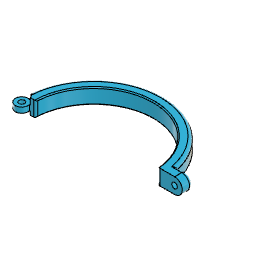
ber_dessus_KOSMOS3-0 (Autodesk Fusion 360 design; units mm, degrees)
Autodesk Fusion 360 part; units mm, degrees
sketch "Esquisse10" plane through (0, 0, 0) normal (0, 0, 1) x (1, 0, 0)
  line L0 (57.7841, 5) -> (81.3781, 5)
  line L1 (81.3781, 5) -> (81.3781, 15)
  line L2 (81.3781, 15) -> (66.325, 15)
  line L3 (-64.0405, 1.5) -> (-57.9806, 1.5)
  line L4 (-58, 0.0001) -> (-58, 0)
  arc A0 (66.325, 15) -> (-67.7547, 5.7709) centre (0, 0) ccw
  arc A1 (57.7841, 5) -> (-57.9806, 1.5) centre (0, 0) ccw
  arc A2 (-58, 0.0001) -> (-58, 0) centre (0, 0) ccw
  line L5 (0, 0) -> (-100, 0) construction
  circle A3 centre (-70.078, 0) radius 6.221
  circle A4 centre (-70.078, 0) radius 6.921
  dimension "d85" = 116
  dimension "d86" = 136
  dimension "d87" = 5
  dimension "d89" = 23.594
  dimension "d93" = 12.078
  dimension "d94" = 10
  dimension "d95" = 1.5
  dimension "d96" = 12.442
  dimension "d113" = 13.842
  constraint coincident A0.centre A1.centre
  constraint horizontal L0
  constraint vertical L1
  constraint horizontal L2
  constraint horizontal L3
  constraint coincident L4.start A1
  constraint concentric A1 A2
  constraint horizontal L5
  constraint coincident L3.start A3
  constraint concentric A3 A4
  measures "d85" diameter of A1
  measures "d86" diameter of A0
  measures "d87" distance of A0.centre L0
  measures "d89" distance of L0.start L0.end
  measures "d93" distance of L4.end A3.centre
  measures "d94" distance of L0 L2
  measures "d95" distance of L3 L5
  measures "d96" diameter of A3
  measures "d113" diameter of A4
extrude "Extrusion9" add sketch "Esquisse10" along normal blind 15 contours L0 L1 L2 L3 A0 A1 A2 A4 | L3 A0 A3 A4 | A3 picked at (-63.6553, 1.8155)
extrude "Extrusion10" cut sketch "Esquisse10" along normal blind 3.4 contours L3 A0 A3 A4 | A3 picked at (-63.6553, 1.8155)
sketch "Esquisse11" plane through (0, 0, 15) normal (0, 0, 1) x (-1, 0, 0)
  line L0 (-57.7841, -5) -> (-81.3781, -5)
  line L1 (-81.3781, -5) -> (-81.3781, -15)
  line L2 (-81.3781, -15) -> (-66.325, -15)
  arc A0 (-66.325, -15) -> (67.7547, -5.7709) centre (0, 0) ccw
  arc A1 (67.7547, -5.7709) -> (64.0405, -1.5) centre (70.078, 0) ccw
  line L3 (64.0405, -1.5) -> (57.9806, -1.5)
  arc A2 (-57.7841, -5) -> (57.9806, -1.5) centre (0, 0) ccw
  circle A3 centre (70.078, 0) radius 6.221
  circle A4 centre (70.078, 0) radius 6.921
  dimension "d101" = 12.442
  dimension "d114" = 13.842
  constraint concentric A1 A3
  constraint concentric A3 A4
  measures "d101" diameter of A3
  measures "d114" diameter of A4
extrude "Extrusion11" cut sketch "Esquisse11" against normal blind 6.4 contours A0 L3 A3 A4 | A1 A3
sketch "Esquisse12" plane through (0, 15, 0) normal (0, 1, 0) x (-1, 0, 0)
  line L0 (-81.3781, 0) -> (-66.325, 0)
  line L1 (-66.325, 0) -> (-66.325, 15)
  line L2 (-66.325, 15) -> (-81.3781, 15)
  line L3 (-81.3781, 15) -> (-81.3781, 0)
  line L4 (-66.325, 15) -> (-81.3781, 0) construction
  line L5 (-66.325, 0) -> (-81.3781, 15) construction
  circle A0 centre (-73.8515, 7.5) radius 2.7
  dimension "d104" = 5.4
  constraint coincident L1.end L2.start
  constraint coincident L0.start L3.end
  constraint coincident L0.end L1.start
  constraint coincident L2.end L3.start
  constraint midpoint L4 A0.centre
  measures "d104" diameter of A0
extrude "Extrusion12" cut sketch "Esquisse12" against normal blind 10 contours A0
fillet "Congé2" radius 7.5 2 edges at (81.3781, 10, 0) (81.3781, 10, 15)
sketch "Esquisse13" plane through (0, 0, 8.6) normal (0, 0, 1) x (-1, 0, 0)
  arc A0 (67.7547, -5.7709) -> (64.0405, -1.5) centre (70.078, 0) ccw
  circle A1 centre (70.078, 0) radius 2.75
  line L0 (64.0405, -1.5) -> (63.3215, -1.5)
  arc A2 (63.3215, -1.5) -> (67.689, -6.4956) centre (70.078, 0) ccw
  arc A3 (67.689, -6.4956) -> (67.7547, -5.7709) centre (0, 0) ccw
  dimension "d109" = 5.5
  constraint concentric A0 A1
  measures "d109" diameter of A1
extrude "Extrusion13" cut sketch "Esquisse13" against normal blind 6 contours A1
chamfer "Chanfrein5" distance 1 angle 45 2 edges at (-1.7528, 57.9735, 15) (-1.7528, 57.9735, 0)
fillet "Congé3" radius 2 2 edges at (-57.9806, 1.5, 7.5) (57.7841, 5, 7.5)
fillet "Congé4" radius 3 5 edges at (-4.3065, 67.8635, 15) (-4.3065, 67.8635, 0) (70.1015, 15, 0) (81.3781, 15, 7.5) (70.1015, 15, 15)
equation "d85 = ( 58 * 2 ) * 1 mm"
equation "d86 = ( 68 * 2 ) * 1 mm"
equation "d96 = ( 6.221 * 2 ) * 1 mm"
equation "d101 = d96"
equation "d113 = d96 + 1.4 mm"
equation "d114 = d113"
